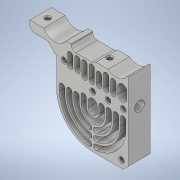
# Autodesk Inventor part: MINI-heatsink
Saved by Autodesk Inventor 2021 (Build 250183000, 183)
## iProperties
Created: 2019-07-10
Material: Všeobecné
Document SubType Name: Modeling
Density: 1 g/cm^3
Appearance: Hliník – leštěný
Project: ORIGINAL PRUSA MINI
Authority: Ing. Robert Turinský
Company: Prusa Development a.s.
Author: Ing. Robert Turinský
Title: MINI-heatsink
Revision Number: R4
Autodesk Inventor part; units mm, degrees
ref_plane "YZ Plane" through (0, 0, 0) normal (1, 0, 0) x (0, 1, 0)
ref_plane "XZ Plane" through (0, 0, 0) normal (0, 1, 0) x (-1, 0, 0)
ref_plane "XY Plane" through (0, 0, 0) normal (0, 0, 1) x (1, 0, 0)
sketch "Náčrt1" plane through (0, 0, 0) normal (0, 0, 1) x (1, 0, 0)
  line L0 (21, -7) -> (11, -7)
  line L1 (11, -7) -> (21, -7)
  line L2 (9, -5) -> (9, -4)
  line L3 (9, -4) -> (6.3443, -4)
  line L4 (-6.3443, -4) -> (-14, -4)
  line L5 (-14, -4) -> (-14, -7)
  arc A0 (29.5, -6) -> (31.3074, -7) centre (34, 0) ccw
  line L6 (29.5, -6) -> (22.7321, -6)
  arc A1 (21, -7) -> (22.7321, -6) centre (21, -5) ccw
  line L7 (9, -5) -> (9, -4)
  line L8 (9, -4) -> (6.3443, -4)
  arc A2 (21, -7) -> (22.7321, -6) centre (21, -5) ccw
  line L9 (22.7321, -6) -> (29.5, -6)
  arc A3 (29.5, -6) -> (31.3074, -7) centre (34, 0) ccw
  arc A4 (9, -5) -> (11, -7) centre (11, -5) ccw
  arc A5 (-6.3443, -4) -> (6.3443, -4) centre (0, 0) ccw
  arc A6 (31.3074, -7) -> (40.3443, -4) centre (34, 0) ccw
  circle A7 centre (38, -21) radius 1.2
  circle A8 centre (21, -21) radius 1.2
  circle A9 centre (29.5, -21) radius 1.2
  circle A10 centre (5, -14) radius 1.2
  circle A11 centre (37, -46) radius 1.2
  line L10 (41, -4) -> (41, -47)
  line L11 (38, -50) -> (21, -50)
  line L12 (1, -30) -> (1, -14)
  line L13 (41, -4) -> (40.3443, -4)
  line L14 (-14, -7) -> (-12, -9)
  line L15 (-12, -9) -> (-4, -9)
  line L16 (-4, -9) -> (1, -14)
  line L17 (36.5, -25) -> (36.5, -30)
  line L18 (39.5, -30) -> (39.5, -25)
  line L19 (35.5, -30) -> (35.5, -25)
  line L20 (32.5, -25) -> (32.5, -30)
  line L21 (31.5, -30) -> (31.5, -25)
  line L22 (28.5, -25) -> (28.5, -30)
  line L23 (27.5, -30) -> (27.5, -25)
  line L24 (24.5, -30) -> (24.5, -25)
  line L25 (18.5, -30) -> (18.5, -26)
  line L26 (17.5, -25) -> (17.5, -30)
  line L27 (14.5, -30) -> (14.5, -25)
  line L28 (13.5, -30) -> (13.5, -25)
  line L29 (10.5, -30) -> (10.5, -25)
  line L30 (9.5, -30) -> (9.5, -27)
  line L31 (6.5, -30) -> (6.5, -27)
  line L32 (5.5, -30) -> (5.5, -27)
  line L33 (23.5, -26) -> (23.5, -30)
  arc A12 (39.5, -25) -> (36.5, -25) centre (38, -25) ccw
  arc A13 (35.5, -25) -> (32.5, -25) centre (34, -25) ccw
  arc A14 (31.5, -25) -> (28.5, -25) centre (30, -25) ccw
  arc A15 (27.5, -25) -> (24.5, -25) centre (26, -25) ccw
  arc A16 (17.5, -25) -> (14.5, -25) centre (16, -25) ccw
  arc A17 (13.5, -25) -> (10.5, -25) centre (12, -25) ccw
  arc A18 (9.5, -27) -> (6.5, -27) centre (8, -27) ccw
  arc A19 (5.5, -27) -> (2.5, -27) centre (4, -27) ccw
  line L34 (2.5, -30) -> (2.5, -27)
  line L35 (34, -17) -> (34, -10.5)
  line L36 (31, -17) -> (31, -10.5)
  line L37 (30, -9.5) -> (30, -17)
  line L38 (27, -17) -> (27, -9.5)
  line L39 (26, -11) -> (26, -17)
  line L40 (23, -11) -> (23, -17)
  line L41 (22, -9.5) -> (22, -17)
  line L42 (19, -17) -> (19, -9.5)
  line L43 (18, -9.5) -> (18, -17)
  line L44 (15, -17) -> (15, -9.5)
  line L45 (14, -9.5) -> (14, -17)
  line L46 (7, -9.5) -> (7, -15)
  line L47 (10, -9) -> (10, -15)
  line L48 (11, -9.5) -> (11, -17)
  arc A20 (35, -16) -> (40, -16) centre (37.5, -16) ccw
  arc A21 (40, -11.5) -> (35, -11.5) centre (37.5, -11.5) ccw
  arc A22 (31, -17) -> (34, -17) centre (32.5, -17) ccw
  arc A23 (10, -9.5) -> (7, -9.5) centre (8.5, -9.5) ccw
  arc A24 (34, -10.5) -> (31, -10.5) centre (32.5, -10.5) ccw
  arc A25 (30, -9.5) -> (27, -9.5) centre (28.5, -9.5) ccw
  arc A26 (14, -9.5) -> (11, -9.5) centre (12.5, -9.5) ccw
  arc A27 (18, -9.5) -> (15, -9.5) centre (16.5, -9.5) ccw
  arc A28 (22, -9.5) -> (19, -9.5) centre (20.5, -9.5) ccw
  arc A29 (26, -11) -> (23, -11) centre (24.5, -11) ccw
  arc A30 (27, -17) -> (30, -17) centre (28.5, -17) ccw
  arc A31 (23, -17) -> (26, -17) centre (24.5, -17) ccw
  arc A32 (19, -17) -> (22, -17) centre (20.5, -17) ccw
  arc A33 (15, -17) -> (18, -17) centre (16.5, -17) ccw
  arc A34 (7, -15) -> (10, -15) centre (8.5, -15) ccw
  arc A35 (11, -17) -> (14, -17) centre (12.5, -17) ccw
  line L49 (35, -11.5) -> (35, -16)
  line L50 (40, -11.5) -> (40, -16)
  arc A36 (1, -30) -> (21, -50) centre (21, -30) ccw
  line L51 (38, -50) -> (41, -47)
  line L52 (20, -30) -> (22, -30)
  line L53 (21, -29) -> (21, -31)
  arc A37 (18.5, -30) -> (23.5, -30) centre (21, -30) ccw
  arc A38 (17.5, -30) -> (24.5, -30) centre (21, -30) ccw
  arc A39 (14.5, -30) -> (27.5, -30) centre (21, -30) ccw
  arc A40 (22.5925, -37.329) -> (28.5, -30) centre (21, -30) ccw
  arc A41 (13.5, -30) -> (19.4075, -37.329) centre (21, -30) ccw
  arc A42 (23.2295, -40.2606) -> (31.5, -30) centre (21, -30) ccw
  arc A43 (10.5, -30) -> (18.7705, -40.2606) centre (21, -30) ccw
  arc A44 (9.5, -30) -> (19.2952, -41.3729) centre (21, -30) ccw
  arc A45 (22.7048, -41.3729) -> (32.5, -30) centre (21, -30) ccw
  arc A46 (23.5, -26) -> (18.5, -26) centre (21, -26) ccw
  arc A47 (23.1495, -44.3398) -> (35.5, -30) centre (21, -30) ccw
  arc A48 (6.5, -30) -> (18.8505, -44.3398) centre (21, -30) ccw
  arc A49 (22.8165, -45.3932) -> (36.5, -30) centre (21, -30) ccw
  arc A50 (5.5, -30) -> (19.1835, -45.3932) centre (21, -30) ccw
  arc A51 (2.5, -30) -> (18.8319, -48.3725) centre (21, -30) ccw
  arc A52 (23.1681, -48.3725) -> (39.5, -30) centre (21, -30) ccw
  arc A53 (22.5925, -37.329) -> (23.2295, -40.2606) centre (22.911, -38.7948) ccw
  arc A54 (22.7048, -41.3729) -> (23.1495, -44.3398) centre (22.9272, -42.8564) ccw
  arc A55 (22.8165, -45.3932) -> (23.1681, -48.3725) centre (22.9923, -46.8829) ccw
  arc A56 (18.8319, -48.3725) -> (19.1835, -45.3932) centre (19.0077, -46.8829) ccw
  arc A57 (18.8505, -44.3398) -> (19.2952, -41.3729) centre (19.0728, -42.8564) ccw
  arc A58 (18.7705, -40.2606) -> (20.0658, -37.6564) centre (19.089, -38.7948) ccw
  arc A59 (20.0658, -37.6564) -> (19.4075, -37.329) centre (19.089, -38.7948) ccw
  arc A60 (18.7705, -40.2606) -> (19.4075, -37.329) centre (19.089, -38.7948) ccw
  point P0 (0, 0)
  constraints: 112 point on circle, 108 end point, 61 centre point
sketch "Náčrt2" plane through (0, 0, 0) normal (0, 0, 1) x (1, 0, 0)
  line L0 (-14, -7) -> (-14, -4)
  line L1 (-14, -4) -> (-6.3443, -4)
  line L2 (6.3443, -4) -> (9, -4)
  line L3 (9, -4) -> (9, -4.5)
  arc A0 (-6.3443, -4) -> (6.3443, -4) centre (0, 0) ccw
  arc A1 (29.5, -6) -> (40.3443, -4) centre (34, 0) ccw
  line L4 (22.7321, -6) -> (29.5, -6)
  line L5 (20.7321, -7) -> (11.5, -7)
  line L6 (40.3443, -4) -> (41, -4)
  line L7 (41, -4) -> (41, -47)
  line L8 (41, -47) -> (38, -50)
  line L9 (38, -50) -> (21, -50)
  arc A2 (1, -30) -> (21, -50) centre (21, -30) ccw
  line L10 (1, -30) -> (1, -14)
  line L11 (1, -14) -> (-4, -9)
  line L12 (-4, -9) -> (-12, -9)
  line L13 (-12, -9) -> (-14, -7)
  circle A3 centre (37, -46) radius 1.25
  circle A4 centre (38, -21) radius 1.25
  circle A5 centre (29.5, -21) radius 1.25
  circle A6 centre (21, -21) radius 1.25
  circle A7 centre (5, -14) radius 1.25
  line L14 (2.5, -27) -> (2.5, -30)
  line L15 (5.5, -30) -> (5.5, -27)
  line L16 (6.5, -27) -> (6.5, -30)
  line L17 (9.5, -27) -> (9.5, -30)
  line L18 (10.5, -30) -> (10.5, -27)
  line L19 (13.5, -27) -> (13.5, -30)
  line L20 (14.5, -30) -> (14.5, -25)
  line L21 (17.5, -25) -> (17.5, -30)
  line L22 (18.5, -30) -> (18.5, -26)
  line L23 (23.5, -26) -> (23.5, -30)
  line L24 (24.5, -30) -> (24.5, -25)
  line L25 (27.5, -25) -> (27.5, -30)
  line L26 (28.5, -30) -> (28.5, -25)
  line L27 (31.5, -25) -> (31.5, -30)
  line L28 (32.5, -30) -> (32.5, -25)
  line L29 (35.5, -25) -> (35.5, -30)
  line L30 (36.5, -30) -> (36.5, -25)
  line L31 (39.5, -25) -> (39.5, -30)
  arc A8 (5.5, -27) -> (2.5, -27) centre (4, -27) ccw
  arc A9 (9.5, -27) -> (6.5, -27) centre (8, -27) ccw
  arc A10 (17.5, -25) -> (14.5, -25) centre (16, -25) ccw
  arc A11 (23.5, -26) -> (18.5, -26) centre (21, -26) ccw
  arc A12 (27.5, -25) -> (24.5, -25) centre (26, -25) ccw
  arc A13 (31.5, -25) -> (28.5, -25) centre (30, -25) ccw
  arc A14 (35.5, -25) -> (32.5, -25) centre (34, -25) ccw
  arc A15 (39.5, -25) -> (36.5, -25) centre (38, -25) ccw
  arc A16 (18.5, -30) -> (23.5, -30) centre (21, -30) ccw
  arc A17 (17.5, -30) -> (24.5, -30) centre (21, -30) ccw
  arc A18 (14.5, -30) -> (27.5, -30) centre (21, -30) ccw
  arc A19 (18.7705, -40.2606) -> (19.4075, -37.329) centre (19.089, -38.7948) ccw
  arc A20 (22.5925, -37.329) -> (23.2295, -40.2606) centre (22.911, -38.7948) ccw
  arc A21 (22.7048, -41.3729) -> (23.1495, -44.3398) centre (22.9272, -42.8564) ccw
  arc A22 (18.8505, -44.3398) -> (19.2952, -41.3729) centre (19.0728, -42.8564) ccw
  arc A23 (18.8319, -48.3725) -> (19.1835, -45.3932) centre (19.0077, -46.8829) ccw
  arc A24 (22.8165, -45.3932) -> (23.1681, -48.3725) centre (22.9923, -46.8829) ccw
  arc A25 (13.5, -30) -> (19.4075, -37.329) centre (21, -30) ccw
  arc A26 (10.5, -30) -> (18.7705, -40.2606) centre (21, -30) ccw
  arc A27 (22.5925, -37.329) -> (28.5, -30) centre (21, -30) ccw
  arc A28 (23.2295, -40.2606) -> (31.5, -30) centre (21, -30) ccw
  arc A29 (22.7048, -41.3729) -> (32.5, -30) centre (21, -30) ccw
  arc A30 (23.1495, -44.3398) -> (35.5, -30) centre (21, -30) ccw
  arc A31 (22.8165, -45.3932) -> (36.5, -30) centre (21, -30) ccw
  arc A32 (23.1681, -48.3725) -> (39.5, -30) centre (21, -30) ccw
  arc A33 (9.5, -30) -> (19.2952, -41.3729) centre (21, -30) ccw
  arc A34 (6.5, -30) -> (18.8505, -44.3398) centre (21, -30) ccw
  arc A35 (5.5, -30) -> (19.1835, -45.3932) centre (21, -30) ccw
  arc A36 (2.5, -30) -> (18.8319, -48.3725) centre (21, -30) ccw
  line L32 (35, -11.5) -> (35, -16)
  line L33 (40, -16) -> (40, -11.5)
  arc A37 (40, -11.5) -> (35, -11.5) centre (37.5, -11.5) ccw
  arc A38 (35, -16) -> (40, -16) centre (37.5, -16) ccw
  arc A39 (34, -10.5) -> (31, -10.5) centre (32.5, -10.5) ccw
  arc A40 (31, -17) -> (34, -17) centre (32.5, -17) ccw
  arc A41 (27, -17) -> (30, -17) centre (28.5, -17) ccw
  arc A42 (30, -9.5) -> (27, -9.5) centre (28.5, -9.5) ccw
  arc A43 (26, -11) -> (23, -11) centre (24.5, -11) ccw
  arc A44 (23, -17) -> (26, -17) centre (24.5, -17) ccw
  arc A45 (19, -17) -> (22, -17) centre (20.5, -17) ccw
  arc A46 (22, -9.5) -> (19, -9.5) centre (20.5, -9.5) ccw
  arc A47 (18, -9.5) -> (15, -9.5) centre (16.5, -9.5) ccw
  arc A48 (15, -17) -> (18, -17) centre (16.5, -17) ccw
  arc A49 (14, -9.5) -> (11, -9.5) centre (12.5, -9.5) ccw
  arc A50 (10, -9.5) -> (7, -9.5) centre (8.5, -9.5) ccw
  arc A51 (7, -15) -> (10, -15) centre (8.5, -15) ccw
  line L34 (34, -10.5) -> (34, -17)
  line L35 (31, -17) -> (31, -10.5)
  line L36 (30, -9.5) -> (30, -17)
  line L37 (27, -17) -> (27, -9.5)
  line L38 (26, -11) -> (26, -17)
  line L39 (23, -17) -> (23, -11)
  line L40 (22, -9.5) -> (22, -17)
  line L41 (19, -17) -> (19, -9.5)
  line L42 (18, -9.5) -> (18, -17)
  line L43 (15, -17) -> (15, -9.5)
  line L44 (14, -9.5) -> (14, -15)
  line L45 (11, -15) -> (11, -9.5)
  line L46 (10, -9.5) -> (10, -15)
  line L47 (7, -15) -> (7, -9.5)
  line L48 (1, -21) -> (10, -21)
  line L49 (13.2814, -24.4) -> (1, -24.4)
  line L50 (10, -21) -> (41, -21)
  line L51 (41, -21) -> (41, -23.25)
  line L52 (41, -23.25) -> (13.7, -23.25)
  arc A52 (13.5, -27) -> (10.5, -27) centre (12, -27) ccw
  arc A53 (11, -15) -> (13.9981, -14.924) centre (12.5, -15) ccw
  line L53 (1, -25.1) -> (1, -21)
  line L54 (1.7, -24.4) -> (1, -24.4)
  line L55 (1, -24.4) -> (1, -25.1)
  line L56 (41, -21) -> (15.1811, -21)
  line L57 (16.182, -23.75) -> (41, -23.75)
  line L58 (41, -23.75) -> (41, -21)
  line L59 (16.0047, -23.263) -> (15.1811, -21)
  arc A54 (17.5, -25.75) -> (14.5, -25.75) centre (16, -25.75) ccw
  arc A55 (23.5, -26.75) -> (18.5, -26.75) centre (21, -26.75) ccw
  arc A56 (27.5, -25.75) -> (24.5, -25.75) centre (26, -25.75) ccw
  arc A57 (31.5, -25.75) -> (28.5, -25.75) centre (30, -25.75) ccw
  arc A58 (35.5, -25.75) -> (32.5, -25.75) centre (34, -25.75) ccw
  arc A59 (39.5, -25.75) -> (36.5, -25.75) centre (38, -25.75) ccw
  arc A60 (35, -15.25) -> (40, -15.25) centre (37.5, -15.25) ccw
  arc A61 (23, -16.25) -> (26, -16.25) centre (24.5, -16.25) ccw
  arc A62 (19, -16.25) -> (22, -16.25) centre (20.5, -16.25) ccw
  arc A63 (15, -16.25) -> (18, -16.25) centre (16.5, -16.25) ccw
  arc A64 (31, -16.25) -> (34, -16.25) centre (32.5, -16.25) ccw
  arc A65 (27, -16.25) -> (30, -16.25) centre (28.5, -16.25) ccw
  line L60 (13.7, -23.25) -> (13.2814, -24.4)
  line L61 (16, -23.25) -> (16.182, -23.75)
  arc A66 (9, -4.5) -> (11.5, -7) centre (11.5, -4.5) ccw
  arc A67 (20.7321, -7) -> (22.7321, -6) centre (20.7321, -4.5) ccw
  point P0 (9, -5)
  point P1 (11, -7)
  point P2 (11, -5)
  point P3 (21, -7)
  point P4 (21, -5)
  point P5 (12.5, -17)
  point P6 (12, -25)
  point P7 (10.5, -25)
  point P8 (13.5, -25)
  dimension "d0" = 2.5
  dimension "d16" = 6.8
  dimension "d17" = 4.5
  dimension "d21" = 8.2
  dimension "d49" = 5.5
  dimension "d50" = 70
  dimension "d51" = 25
  dimension "d52" = 0.5
  dimension "d55" = 0.5
  dimension "d56" = 3.25
  dimension "d57" = 3.25
  dimension "d133" = 70
  dimension "d134" = 70
  dimension "d135" = 2.3
  dimension "d136" = 12.7
  dimension "d146" = 2.5
  constraints: 127 point on circle, 124 end point, 68 centre point, 55 coincident, 49 tangent, 34 point on line, 26 equal radius, 22 vertical, 15 parallel, 10 horizontal alignment, 5 horizontal, 5 perpendicular, 2 collinear, 2 vertical alignment
  measures "d0" diameter of A3
  measures "d16" diameter of L49 L48
  measures "d17" diameter of L52 L50
  measures "d21" diameter of L53.start L48
  measures "d49" diameter of L57 L50
  measures "d50" angle of L50 L59
  measures "d51" distance of L59.start L57.end
  measures "d52" distance edge to line of A54 L57
  measures "d55" distance edge to line of A55 L57
  measures "d56" distance edge to line of A63 L50
  measures "d57" distance edge to line of A60 L56
  measures "d133" angle of L50 L60
  measures "d134" angle of L56 L61
  measures "d135" distance of L52.end L61.start
  measures "d136" distance from line of L10 L52.end
  measures "d146" radius of A66
extrude "Vysunutí1" add sketch "Náčrt2" along normal mid plane 12 contours L0 L1 A0 L2 L3 A66 L5 A67 L4 A1 L6 L7 L50 A4 A5 A6 L48 L10 L11 L12 L13 | L48 L50 L59 L52 L60 L49 L10 | L49 L60 L52 L59 L61 A10 L20 A18 L25 A12 L57 A13 L26 A27 A20 A28 L27 A14 L28 A29 A21 A30 L29 A15 L30 A31 A24 A32 L31 L7 L8 L9 A2 L10 | L50 A6 A5 A4 L7 L52 L59 | L52 L7 L57 A15 A14 A13 A12 A11 A10 L61 L59 | L57 A11 L22 A16 L23 A12 L24 A17 L21 A10
sketch "Náčrt3" plane through (-14, -4, 6) normal (0, 1, 0) x (1, 0, 0)
  line L0 (14, 14.4) -> (14, -2.4) projected
  line L1 (-11.3985, 6) -> (68.3913, 6) projected
  point P0 (14, 6)
  point P1 (4, 6)
  point P2 (38.5, 6)
  dimension "d4" = 34.5
  dimension "d5" = 10
  constraints: 2 point on line
  measures "d4" distance of point (38.5, 6) point (4, 6)
  measures "d5" distance of point (14, 6) point (4, 6)
hole "Díra1" at (-10, -4, 0) at (24.5, -4, 0) direction (0, -1, 0) diameter 2.5 depth 12 tip angle 118
extrude "Vysunutí2" add sketch "Náčrt2" against normal blind 6 contours L50 A6 | A6 L50 | L50 A5 | A5 L50 | L50 A4 | A4 L50
extrude "Vysunutí4" add sketch "Náčrt2" along normal mid plane 12 contours L61 L57 A10 L21 A54 L20 | A10 L57 L61 | L57 A15 | A15 L31 A59 L30 L57 | L57 A11 L23 A55 L22 | A11 L57 | L57 A14 | A14 L29 A58 L28 L57 | L57 A12 L25 A56 L24 | A12 L57 | L57 A13 | A13 L27 A57 L26 L57 | A60 L33 A38 L32 | L34 A40 L35 A64 | L37 A65 L36 A41 | L38 A44 L39 A61 | L41 A62 L40 A45 | L42 A48 L43 A63
revolve "Rotace1" cut sketch "Náčrt2" angle 360 about axis through (10, -21, 0) along (1, 0, 0) picked at (20.7633, -21.7302) picked at (29.2633, -21.7302) picked at (38.381, -21.2933) contours L48 L50 L59 L52 L60 L49 L10 | L50 A6 A5 A4 L7 L52 L59 | L50 A6 | L52 L7 L57 A15 A14 A13 A12 A11 A10 L61 L59 | L50 A5 | A10 L57 L61 | A4 L50 | L57 A15 | A11 L57 | L57 A14 | A12 L57 | L57 A13
thread "Závit3" size "M3x0.5" class "6H" standard "ANSI Metric M Profile" full length
thread "Závit4" size "M3x0.5" class "6H" standard "ANSI Metric M Profile" full length
thread "Závit5" size "M3x0.5" class "6H" standard "ANSI Metric M Profile" full length
thread "Závit6" size "M3x0.5" class "6H" standard "ANSI Metric M Profile" full length
thread "Závit8" size "M3x0.5" class "6H" standard "ANSI Metric M Profile" full length
thread "Závit9" size "M3x0.5" class "6H" standard "ANSI Metric M Profile" full length
thread "Závit7" size "M3x0.5" class "6H" standard "ANSI Metric M Profile" full length
chamfer "Zkosení1" distance 0.4 angle 45 9 edges at (35.75, -46, 6) (36.75, -21, 6) (28.25, -21, 6) (19.75, -21, 6) (3.75, -14, 6) (-10, -4, -1.25) (24.5, -6, -1.25) (35.75, -46, -6) (3.75, -14, -6)
thread "Závit11" size "M8x1.25" class "6H" standard "ANSI Metric M Profile" length 9
chamfer "Zkosení3" distance 1.25 angle 45 1 edges at (1, -17.6, 0)
fillet "Zaoblení1" radius 2.5 2 edges at (-4, -9, 0) (1, -14, 0)
sketch "Náčrt5" plane through (21, -50, 6) normal (0, -1, 0) x (1, 0, 0)
  line L0 (17, 0) -> (20, 0) projected
  line L1 (17, -12) -> (17, 0) projected
  line L2 (-5.9842, -9.375) -> (-5.9842, -2.625) construction
  line L3 (-5.9842, -2.625) -> (16.5, -2.625) construction
  line L4 (16.5, -2.625) -> (16.5, -9.375) construction
  line L5 (16.5, -9.375) -> (-5.9842, -9.375) construction
  line L6 (20, -12) -> (20, 0) projected
  point P0 (-21, -6)
  point P1 (15.5418, -5.5333)
  point P2 (15.5418, -2.7333)
  dimension "d103" = 2.8
  dimension "d114" = 3.5
  dimension "d121" = 6.75
  dimension "d130" = 2.625
  constraints: 1 horizontal, 1 vertical alignment, 2 other
  measures "d103" distance of point (15.542, -5.533) point (15.542, -2.733)
  measures "d114" distance between parallel lines of L6 L4
  measures "d121" distance of L3.end L4.end
  measures "d130" distance between parallel lines of L0 L3
sketch "Náčrt6" plane through (41, -47, 6) normal (1, 0, 0) x (0, 0, -1)
  circle A0 centre (6, 26) radius 2.75 projected
  line L0 (12, 43) -> (0, 43) projected
  line L1 (0, 0) -> (0, 43) projected
  line L2 (12, 0) -> (0, 0) projected
  line L3 (12, 43) -> (12, 0) projected
  line L4 (1, 11) -> (11, 11) construction
  line L5 (11, 11) -> (11, 1) construction
  line L6 (11, 1) -> (1, 1) construction
  line L7 (1, 1) -> (1, 11) construction
  point P0 (6, 47)
  dimension "d87" = 10
  dimension "d95" = 1
  dimension "d96" = 1
  constraints: 1 horizontal, 2 other
  measures "d87" distance of L5.end L6.end
  measures "d95" distance between parallel lines of L1 L7
  measures "d96" distance between parallel lines of L2 L6
equation "\"d50\" = d133"
equation "\"d55\" = d52"
equation "\"d56\" = 0.5 * d49 + d52"
equation "\"d57\" = d56"
equation "\"d134\" = d133"
equation "\"d6\" = d0"
equation "\"d13\" = 0.5 * d2"
equation "\"d58\" = d2"
equation "\"d130\" = -0.5 * d121 + 0.5 * d2"
equation "\"d95\" = -0.5 * d87 + 0.5 * d2"
equation "\"d96\" = d95"
equation "\"d2\" = 12"
